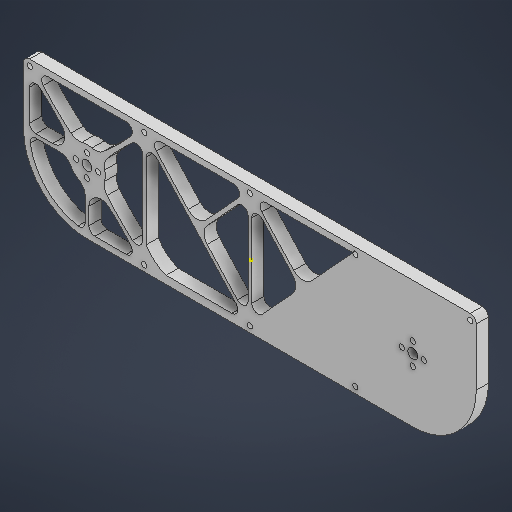
# Autodesk Inventor part: кб 2025-2026
Saved by Autodesk Inventor 2025 (Build 290162000, 162)
## iProperties
Created: 2025-09-02
Part Number: кб 2025-2026
Material: Типовые
Document SubType Name: Modeling
Designer: Phantom
Density: 1 g/cm^3
Appearance: По умолчанию
Author: Phantom
Autodesk Inventor part; units mm, degrees
ref_plane "YZ Plane" through (0, 0, 0) normal (1, 0, 0) x (0, 1, 0)
ref_plane "XZ Plane" through (0, 0, 0) normal (0, 1, 0) x (-1, 0, 0)
ref_plane "XY Plane" through (0, 0, 0) normal (0, 0, 1) x (1, 0, 0)
sketch "Эскиз1" plane through (0, 0, 0) normal (0, 0, 1) x (1, 0, 0)
  arc A0 (132.2862, -52.3121) -> (184.2862, -0.3121) centre (132.2862, -0.3121) ccw
  line L0 (-134.5611, -52.3121) -> (132.2862, -52.3121)
  line L1 (-186.5611, -0.3121) -> (-186.5611, 46.6879)
  line L2 (184.2862, -0.3121) -> (184.2862, 46.6879)
  line L3 (-134.5611, 51.6879) -> (-181.5611, 51.6879)
  line L4 (-181.5611, 51.6879) -> (179.2862, 51.6879)
  arc A1 (-186.5611, -0.3121) -> (-134.5611, -52.3121) centre (-134.5611, -0.3121) ccw
  circle A2 centre (-134.5611, -0.3121) radius 4
  circle A3 centre (-134.5611, 8.6879) radius 2.1
  circle A4 centre (-143.5611, -0.3121) radius 2.1
  circle A5 centre (-134.5611, -9.3121) radius 2.1
  circle A6 centre (-125.5611, -0.3121) radius 2.1
  circle A7 centre (132.2862, -0.3121) radius 4
  circle A8 centre (132.2862, 8.6879) radius 2.1
  circle A9 centre (123.2862, -0.3121) radius 2.1
  circle A10 centre (132.2862, -9.3121) radius 2.1
  circle A11 centre (141.2862, -0.3121) radius 2.1
  arc A12 (-181.5611, 51.6879) -> (-186.5611, 46.6879) centre (-181.5611, 46.6879) ccw
  arc A13 (184.2862, 46.6879) -> (179.2862, 51.6879) centre (179.2862, 46.6879) ccw
  circle A14 centre (-181.5611, 46.6879) radius 2.1
  circle A15 centre (179.2862, 46.6879) radius 2.1
  circle A16 centre (-87.5611, -47.3121) radius 2.1
  circle A17 centre (85.2862, -47.3121) radius 2.1
  circle A18 centre (-1.1374, -47.3121) radius 2.1
  circle A19 centre (-1.1374, 46.6879) radius 2.1
  circle A20 centre (-87.5611, 46.6879) radius 2.1
  circle A21 centre (85.2862, 46.6879) radius 2.1
  line L5 (179.2862, 44.5879) -> (179.2862, -0.3121)
  arc A22 (-181.5611, 51.6879) -> (-186.5611, 46.6879) centre (-181.5611, 46.6879) ccw
  line L6 (-181.5611, 44.5879) -> (-181.5611, -0.3121)
  arc A23 (-181.5611, -0.3121) -> (-134.5611, -47.3121) centre (-134.5611, -0.3121) ccw
  arc A24 (-164.0709, -36.8931) -> (-134.5611, -47.3121) centre (-134.5611, -0.3121) ccw
  arc A25 (-132.8051, -9.1391) -> (-132.4754, -9.0671) centre (-134.5611, -0.3121) ccw
  line L7 (-80.49, 46.6879) -> (-80.6353, 46.5425)
  line L8 (-174.49, 46.6879) -> (-89.6611, 46.6879)
  line L9 (-179.4611, 46.6879) -> (-94.6321, 46.6879)
  line L10 (-80.49, 46.6879) -> (-3.2374, 46.6879)
  line L11 (-85.4611, 46.6879) -> (-7.9295, 46.6879)
  line L12 (5.6547, 46.6879) -> (78.4941, 46.6879)
  line L13 (0.9626, 46.6879) -> (83.1862, 46.6879)
  line L14 (87.3862, 46.6879) -> (172.2152, 46.6879)
  line L15 (92.3573, 46.6879) -> (177.1862, 46.6879)
  arc A26 (132.2862, -47.3121) -> (179.2862, -0.3121) centre (132.2862, -0.3121) ccw
  arc A27 (168.8672, -29.822) -> (179.2862, -0.3121) centre (132.2862, -0.3121) ccw
  line L16 (-89.6611, -47.3121) -> (-134.5611, -47.3121)
  line L17 (-80.6353, -47.1668) -> (-80.49, -47.3121)
  line L18 (5.6547, -47.3121) -> (85.2862, -47.3121)
  line L19 (132.2862, -47.3121) -> (0.9626, -47.3121)
  line L20 (-7.9295, -47.3121) -> (-80.769, -47.3121)
  line L21 (-85.4611, -47.3121) -> (-3.2374, -47.3121)
  point P0 (-186.5611, 44.6168)
  point P1 (-75.49, 51.6879)
  point P2 (-1.1374, 46.6879)
  dimension "d2" = 8
  dimension "d4" = 4.2
  dimension "d7" = 360
  dimension "d13" = 4.2
  dimension "d14" = 360
  dimension "d15" = 5
  dimension "d17" = 4.2
  dimension "d19" = 4.2
  dimension "d21" = 4.2
  dimension "d23" = 4.2
  dimension "d35" = 99
  constraints: 44 end point, 35 point on circle, 27 centre point, 14 point on line, 10 tangent, 5 coincident, 1 equal radius, 1 horizontal, 1 vertical, 21 other
  measures "d2" diameter of A2
  measures "d4" diameter of A3
  measures "d13" diameter of A8
  measures "d15" radius of A12
  measures "d17" diameter of A14
  measures "d19" diameter of A15
  measures "d21" diameter of A16
  measures "d23" diameter of A19
  measures "d35" distance from line of L1 A16.centre
extrude "Выдавливание1" add sketch "Эскиз1" along normal blind 10 contours L0 A1 L1 A12 L3 L4 A13 L2 A0 | L9 L8 A20 L11 L10 A19 L13 L12 A21 L14 L15 A15 L5 A26 L19 A17 L18 A18 L21 L20 A16 L16 A23 L6 A14
sketch "Эскиз2" plane through (0, 0, 10) normal (0, 0, 1) x (1, 0, 0)
  arc A0 (-186.5611, -0.3121) -> (-134.5611, -52.3121) centre (-134.5611, -0.3121) ccw projected
  circle A1 centre (-143.5611, -0.3121) radius 2.1 projected
  circle A2 centre (-181.5611, 46.6879) radius 2.1 projected
  circle A3 centre (-87.5611, 46.6879) radius 2.1 projected
  line L0 (-181.5611, 46.6879) -> (-102.4688, 46.6879)
  circle A4 centre (-1.1374, -47.3121) radius 2.1 projected
  line L1 (-1.1374, -47.3121) -> (-87.5611, -47.3121)
  circle A5 centre (-134.5611, -0.3121) radius 15
  circle A6 centre (-87.5611, 46.6879) radius 5
  circle A7 centre (-181.5611, 46.6879) radius 5
  circle A8 centre (-87.5611, -47.3121) radius 5
  circle A9 centre (-1.1374, -47.3121) radius 5
  circle A10 centre (-1.1374, 46.6879) radius 5
  line L2 (179.2862, 51.6879) -> (-181.5611, 51.6879) projected
  arc A11 (-181.5611, 51.6879) -> (-186.5611, 46.6879) centre (-181.5611, 46.6879) ccw projected
  line L3 (-186.5611, 46.6879) -> (-186.5611, -0.3121) projected
  arc A12 (-186.5611, -0.3121) -> (-134.5611, -52.3121) centre (-134.5611, -0.3121) ccw projected
  line L4 (-134.5611, -52.3121) -> (132.2862, -52.3121) projected
  arc A13 (132.2862, -52.3121) -> (184.2862, -0.3121) centre (132.2862, -0.3121) ccw projected
  line L5 (184.2862, -0.3121) -> (184.2862, 46.6879) projected
  arc A14 (184.2862, 46.6879) -> (179.2862, 51.6879) centre (179.2862, 46.6879) ccw projected
  circle A15 centre (85.2862, -47.3121) radius 2.1 projected
  circle A16 centre (179.2862, 46.6879) radius 2.1 projected
  circle A17 centre (85.2862, 46.6879) radius 2.1 projected
  circle A18 centre (-1.1374, 46.6879) radius 2.1 projected
  circle A19 centre (-87.5611, 46.6879) radius 2.1 projected
  circle A20 centre (-181.5611, 46.6879) radius 2.1 projected
  circle A21 centre (-87.5611, -47.3121) radius 2.1 projected
  circle A22 centre (123.2862, -0.3121) radius 2.1 projected
  circle A23 centre (132.2862, 8.6879) radius 2.1 projected
  circle A24 centre (-125.5611, -0.3121) radius 2.1 projected
  circle A25 centre (-134.5611, -9.3121) radius 2.1 projected
  circle A26 centre (-134.5611, 8.6879) radius 2.1 projected
  circle A27 centre (-1.1374, -47.3121) radius 2.1 projected
  circle A28 centre (132.2862, -0.3121) radius 4 projected
  circle A29 centre (132.2862, -9.3121) radius 2.1 projected
  circle A30 centre (141.2862, -0.3121) radius 2.1 projected
  circle A31 centre (-143.5611, -0.3121) radius 2.1 projected
  circle A32 centre (-134.5611, -0.3121) radius 4 projected
  line L6 (179.2862, 46.6879) -> (179.2862, -0.3121)
  arc A33 (132.2862, -47.3121) -> (179.2862, -0.3121) centre (132.2862, -0.3121) ccw
  line L7 (-102.4787, -47.3121) -> (-128.0611, -47.3121)
  arc A34 (-180.9948, -7.5859) -> (-141.8349, -46.7458) centre (-134.5611, -0.3121) ccw
  line L8 (-181.5611, 6.1879) -> (-181.5611, 31.7702)
  line L9 (-88.1824, -48.8121) -> (-1.1374, -48.8121)
  line L10 (-180.0761, 45.203) -> (-181.5611, 46.6879)
  arc A35 (-181.5611, 6.1879) -> (-176.5611, 1.1879) centre (-176.5611, 6.1879) ccw
  arc A36 (-176.055, -1.8121) -> (-180.9948, -7.5859) centre (-176.055, -6.8121) ccw
  arc A37 (-141.8349, -46.7458) -> (-136.0611, -41.8061) centre (-141.0611, -41.8061) ccw
  arc A38 (-133.0611, -42.3121) -> (-128.0611, -47.3121) centre (-128.0611, -42.3121) ccw
  line L11 (85.2862, 46.6879) -> (85.2862, -47.3121)
  line L12 (85.2862, 46.6879) -> (-1.1374, -47.3121)
  line L13 (-87.5611, 41.6879) -> (-87.5611, -32.3944)
  line L14 (-133.0611, -15.2369) -> (-133.0611, -42.3121)
  line L15 (-134.5611, -15.3121) -> (-134.5611, -47.3121)
  line L16 (-136.0611, -15.2369) -> (-136.0611, -41.8061)
  line L17 (-149.4859, -1.8121) -> (-176.055, -1.8121)
  line L18 (-149.5611, -0.3121) -> (-181.5611, -0.3121)
  line L19 (-149.4859, 1.1879) -> (-176.5611, 1.1879)
  arc A39 (-126.2901, 12.2015) -> (-98.6785, 38.427) centre (-242.2895, 161.9803) ccw
  arc A40 (-97.3626, 34.2305) -> (-122.0474, 7.9589) centre (27.7313, -108.0406) ccw
  arc A41 (-147.0747, 7.9589) -> (-173.2978, 35.5585) centre (-297.8894, -109.0766) ccw
  arc A42 (-170.4316, 38.4246) -> (-142.832, 12.2015) centre (-25.7966, 163.0162) ccw
  arc A43 (-98.6905, -39.0488) -> (-126.2901, -12.8257) centre (-243.3255, -163.6405) ccw
  arc A44 (-122.0474, -8.5831) -> (-97.3647, -34.8414) centre (28.7673, 108.4524) ccw
  arc A45 (-166.6434, 46.6879) -> (-170.4316, 38.4246) centre (-166.6434, 41.6879) ccw
  arc A46 (-98.6785, 38.427) -> (-102.4688, 46.6879) centre (-102.4688, 41.6879) ccw
  arc A47 (-173.2978, 35.5585) -> (-181.5611, 31.7702) centre (-176.5611, 31.7702) ccw
  arc A48 (-102.4787, -47.3121) -> (-98.6905, -39.0488) centre (-102.4787, -42.3121) ccw
  line L20 (-84.177, 43.0071) -> (-1.1374, -47.3121)
  line L21 (-87.5611, 46.6879) -> (-85.4611, 46.6879)
  line L22 (-82.5611, 46.6879) -> (-14.5641, 46.6879)
  line L23 (-166.6434, 46.6879) -> (-85.4611, 46.6879)
  line L24 (12.2893, 46.6879) -> (179.2862, 46.6879)
  line L25 (-77.3803, 33.3984) -> (-12.2625, -37.428)
  line L26 (-77.8151, 38.3038) -> (-11.3182, -34.0226)
  line L27 (-87.5611, -47.3121) -> (-87.5611, -45.2121)
  line L28 (-87.5611, -42.3121) -> (-87.5611, 31.6458)
  line L29 (-86.9397, -45.8121) -> (-86.0914, -45.8121)
  line L30 (-82.7914, -45.8121) -> (-15.9432, -45.8121)
  arc A49 (-15.9432, -45.8121) -> (-12.2625, -37.428) centre (-15.9432, -40.8121) ccw
  line L31 (-89.0611, 30.4755) -> (-89.0611, -31.0883)
  line L32 (-86.0611, 30.0143) -> (-86.0611, -32.3944)
  arc A50 (-89.0611, 30.4755) -> (-97.3626, 34.2305) centre (-94.0611, 30.4755) ccw
  arc A51 (-97.3647, -34.8414) -> (-89.0611, -31.0883) centre (-94.0611, -31.0883) ccw
  arc A52 (-77.3803, 33.3984) -> (-86.0611, 30.0143) centre (-81.0611, 30.0143) ccw
  arc A53 (-86.0611, -1.1901) -> (-86.4175, -1.8121) centre (-59.5558, -16.7923) ccw
  arc A54 (-86.0611, -32.3944) -> (-69.7443, -45.8121) centre (-59.5558, -16.7923) ccw
  line L33 (-1.1374, 46.6879) -> (-2.5587, 45.142)
  line L34 (-4.5215, 43.0071) -> (-43.3304, 0.796)
  line L35 (-1.1374, 46.6879) -> (0.2839, 45.142)
  line L36 (2.2467, 43.0071) -> (42.0744, -0.3121)
  line L37 (-11.3182, 33.3984) -> (-42.3116, -0.3121)
  line L38 (9.0433, 33.3984) -> (40.9702, -1.3273)
  line L39 (8.6085, 38.3038) -> (43.1786, 0.7031)
  line L40 (-0.0332, -48.3273) -> (83.7862, 42.8401)
  line L41 (83.7862, 42.8401) -> (83.7862, -47.3121)
  line L42 (9.0433, -34.0226) -> (83.2486, 46.6879)
  line L43 (86.7862, 46.6879) -> (86.7862, -47.3121)
  line L44 (-1.1374, 46.6879) -> (-1.1374, 44.5879)
  line L45 (-1.1374, 41.6879) -> (-1.1374, -32.27)
  line L46 (-2.6374, 30.0143) -> (-2.6374, -30.6385)
  line L47 (0.3626, 30.0143) -> (0.3626, -30.6385)
  arc A55 (-11.3182, -34.0226) -> (-2.6374, -30.6385) centre (-7.6374, -30.6385) ccw
  arc A56 (0.3626, -30.6385) -> (9.0433, -34.0226) centre (5.3626, -30.6385) ccw
  line L48 (-10.8834, 38.3038) -> (-44.3492, 1.9041)
  line L49 (-45.368, 0.796) -> (-45.4535, 0.7031)
  arc A57 (-74.1343, 46.6879) -> (-77.8151, 38.3038) centre (-74.1343, 41.6879) ccw
  arc A58 (-10.8834, 38.3038) -> (-14.5641, 46.6879) centre (-14.5641, 41.6879) ccw
  arc A59 (12.2893, 46.6879) -> (8.6085, 38.3038) centre (12.2893, 41.6879) ccw
  arc A60 (-2.6374, 30.0143) -> (-11.3182, 33.3984) centre (-7.6374, 30.0143) ccw
  arc A61 (9.0433, 33.3984) -> (0.3626, 30.0143) centre (5.3626, 30.0143) ccw
  point P0 (0, 0)
  point P1 (-177.1277, 44.3759)
  point P2 (-181.5611, 41.6879)
  point P3 (-92.5611, -47.3121)
  point P4 (-92.5611, 46.6879)
  point P5 (-176.5611, 46.6879)
  point P6 (-82.5611, -47.3121)
  point P7 (-82.7914, -48.8121)
  point P8 (-144.0538, 11.302)
  point P9 (-82.5611, -47.3121)
  point P10 (-6.1374, -47.3121)
  point P11 (-88.2682, 41.7381)
  point P12 (-122.0474, 7.9589)
  point P13 (-87.5611, 41.6879)
  point P14 (-122.0474, -8.5831)
  point P15 (-88.2682, -42.3624)
  point P16 (-92.5108, -46.605)
  point P17 (-126.2901, -12.8257)
  point P18 (-89.0611, -41.7437)
  point P19 (-83.2286, 44.1919)
  point P20 (-5.4699, 44.1919)
  point P21 (-3.2614, 42.1614)
  point P22 (0.9866, 42.1614)
  point P23 (3.195, 44.1919)
  point P24 (-2.6374, 41.9182)
  point P25 (0.3626, 41.9182)
  point P26 (42.0744, 1.9041)
  point P27 (83.1873, 46.6212)
  point P28 (83.1862, 46.6879)
  point P29 (3.8626, 46.6879)
  point P30 (40.0368, -0.3121)
  point P31 (-6.1374, 46.6879)
  point P32 (87.3862, 46.6879)
  point P33 (-74.1343, 46.6879)
  dimension "d44" = 30
  dimension "d46" = 10
  dimension "d49" = 10
  dimension "d45" = 10
  dimension "d47" = 10
  dimension "d48" = 10
  dimension "d60" = 5
  dimension "d61" = 5
  dimension "d66" = 5
  dimension "d67" = 1.5
  dimension "d68" = 1.5
  dimension "d70" = 5
  dimension "d71" = 1.5
  dimension "d72" = 1.5
  dimension "d73" = 5
  dimension "d74" = 5
  dimension "d76" = 1.5
  dimension "d77" = 1.5
  dimension "d78" = 1.5
  dimension "d79" = 1.5
  dimension "d80" = 1.5
  dimension "d82" = 1.5
  dimension "d83" = 1.5
  dimension "d84" = 5
  dimension "d86" = 5
  constraints: 92 end point, 72 point on circle, 39 tangent, 32 centre point, 27 point on line, 17 parallel, 9 equal radius, 8 perpendicular, 6 coincident, 2 midpoint, 1 horizontal, 1 horizontal alignment, 1 vertical, 34 other
  measures "d45" diameter of A6
  measures "d47" diameter of A8
  measures "d48" diameter of A9
  measures "d60" radius of A35
  measures "d61" radius of A36
  measures "d66" radius of A45
  measures "d67" distance between parallel lines of L20 L25
  measures "d68" distance between parallel lines of L20 L26
  measures "d70" radius of A49
  measures "d71" distance between parallel lines of L13 L31
  measures "d72" distance between parallel lines of L13 L32
  measures "d73" radius of A50
  measures "d74" radius of A51
  measures "d76" distance between parallel lines of L34 L37
  measures "d77" distance between parallel lines of L36 L38
  measures "d78" distance between parallel lines of L36 L39
  measures "d79" distance between parallel lines of L12 L40
  measures "d80" distance between parallel lines of L12 L42
  measures "d82" distance between parallel lines of L45 L46
  measures "d83" distance between parallel lines of L45 L47
  measures "d84" radius of A55
  measures "d86" radius of A57
extrude "Выдавливание2" cut sketch "Эскиз2" against normal blind 10 contours L0 A46 A39 A5 A42 A45 | L22 A58 L48 L26 A57 | A5 L19 A35 L8 A47 A41 | A40 A50 L31 A51 A44 A5 | L39 A59 L24 A17 L42 | L12 L11 A17 | A17 L42 L24 L12 | L11 L24 L43 A17 | A17 L24 L42 | A5 L16 A37 A34 A36 L17 | L24 A17 | L43 L24 A17 | A43 A48 L7 A38 L14 A5 | L25 A49 L30 A54 L32 A52 | L37 A60 L46 A55 L26 | L38 L42 A56 L47 A61
fillet "Сопряжение1" radius 10 14 edges at (-126.2901, 12.2015, 5) (-122.0474, 7.9589, 5) (-142.832, 12.2015, 5) (-147.0747, 7.9589, 5) (-122.0474, -8.5831, 5) (-126.2901, -12.8257, 5) (-133.0611, -15.2369, 5) (-136.0611, -15.2369, 5) (-149.4859, -1.8121, 5) (-149.4859, 1.1879, 5) (-44.3492, 1.9041, 5) (-42.3116, -0.3121, 5) (40.0368, -0.3121, 5) (42.0744, 1.9041, 5)
sketch "Эскиз3" plane through (0, 0, 10) normal (0, 0, 1) x (1, 0, 0)
  point P0 (0, 0)
